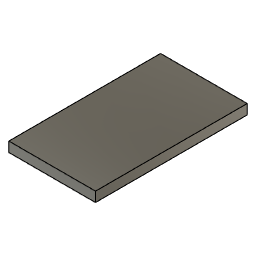
Battery (Autodesk Fusion 360 design; units mm, degrees)
Autodesk Fusion 360 part; units mm, degrees
box "BoxPrimitive2" add length 77 width 44 height 5 placed x (0, 1, 0) y (-1, 0, 0) z (0, 0, 1) at (44, 0, 0)
